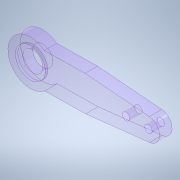
# Autodesk Inventor part: 後ろウィング中間ver2根元
Saved by Autodesk Inventor 2020.2 (Build 242310000, 310)
## iProperties
Created: 2020-05-07
Part Number: 後ろウィング中間ver2根元
Material: ポリカーボネート、クリア
Document SubType Name: Modeling
Designer: mozar
Density: 1.2 g/cm^3
Appearance: ポリカーボネート - クリア
Author: mozar
Autodesk Inventor part; units mm, degrees
ref_plane "YZ Plane" through (0, 0, 0) normal (1, 0, 0) x (0, 1, 0)
ref_plane "XZ Plane" through (0, 0, 0) normal (0, 1, 0) x (-1, 0, 0)
ref_plane "XY Plane" through (0, 0, 0) normal (0, 0, 1) x (1, 0, 0)
sketch "スケッチ1" plane through (0, 0, 0) normal (0, 0, 1) x (1, 0, 0)
  line L0 (-101.5, 47.999998) -> (108.5, 47.999998)
  circle A0 centre (111.885049, -39.000002) radius 4
  circle A1 centre (191.876682, -37.842982) radius 4
  circle A2 centre (111.885049, -39.000002) radius 7
  circle A3 centre (191.876682, -37.842982) radius 7
  line L1 (191.876682, -37.842982) -> (111.885049, -39.000002) construction
  line L2 (191.775442, -30.843714) -> (111.78381, -32.000734)
  line L3 (111.986288, -45.99927) -> (191.977921, -44.84225)
  arc A4 (191.977921, -44.84225) -> (191.775442, -30.843714) centre (191.876682, -37.842982) ccw
  arc A5 (111.78381, -32.000734) -> (111.986288, -45.99927) centre (111.885049, -39.000002) ccw
  line L4 (193.542302, -31.044032) -> (241.704818, -42.842982)
  circle A6 centre (234.566446, -71.981335) radius 30
  line L5 (262.587356, -82.697145) -> (213.725294, -50.402494)
  line L6 (213.725294, -50.402494) -> (190.211062, -44.641931)
  line L7 (264.566446, -121.542906) -> (264.566446, -63.2267)
  line L8 (111.885049, -39.000002) -> (111.885049, 40.999998) construction
  line L9 (118.885049, -39.000002) -> (118.885049, 40.999998)
  line L10 (104.885049, 40.999998) -> (104.885049, -39.000002)
  arc A7 (104.885049, -39.000002) -> (118.885049, -39.000002) centre (111.885049, -39.000002) ccw
  arc A8 (118.885049, 40.999998) -> (104.885049, 40.999998) centre (111.885049, 40.999998) ccw
  circle A9 centre (58.238326, 51.481995) radius 30
  line L11 (113.558078, 34.202868) -> (65.408448, 22.351438)
  line L12 (28.441083, 47.999998) -> (86.70408, 42.010942)
  line L13 (86.70408, 42.010942) -> (110.21202, 47.797128)
  circle A10 centre (113.5, -20.000002) radius 68
  line L14 (315.327237, -100.585467) -> (70.600424, 104.764712)
  line L15 (253.850074, -49.000002) -> (111.885049, -39.000002)
  arc A11 (93.592427, -27.104845) -> (135.370976, -5.924402) centre (95.060351, 21.794105) ccw
  arc A12 (135.370976, -5.924402) -> (135.847591, -3.671647) centre (132.898992, -4.224609) ccw
  arc A13 (135.847591, -3.671647) -> (83.183341, 18.55647) centre (102.157897, -9.989602) ccw
  line L16 (111.885049, -39.000002) -> (112.74718, 40.995353) construction
  line L17 (118.884642, -39.075438) -> (119.746773, 40.919916)
  line L18 (105.747586, 41.070789) -> (104.885455, -38.924565)
  arc A14 (104.885455, -38.924565) -> (118.884642, -39.075438) centre (111.885049, -39.000002) ccw
  arc A15 (119.746773, 40.919916) -> (105.747586, 41.070789) centre (112.74718, 40.995353) ccw
  line L19 (164.994898, 47.999998) -> (164.994898, 25.999998)
  line L20 (164.994898, 25.999998) -> (327.494898, -102.000002)
  circle A16 centre (116.292557, -40.000002) radius 68
  circle A17 centre (-98.885049, -0.000002) radius 67.5
  line L21 (321.363327, -8.500986) -> (-152.668056, 78.49822)
  line L22 (104.889695, -3) -> (104.889695, 0)
  line L23 (104.889695, -3) -> (64.444342, -3)
  line L24 (72.06562, 0) -> (104.889695, 0)
  circle A18 centre (83.376901, -17.5) radius 13.85
  line L25 (198.510163, -35.607603) -> (190.779084, -12.665641)
  line L26 (185.2432, -40.07836) -> (169.408184, 6.912016)
  circle A19 centre (197.837392, 16.492211) radius 30
  line L27 (190.779084, -12.665641) -> (191.876682, 45.89408)
  circle A20 centre (191.876682, -37.842982) radius 83.737062
  line L28 (191.876682, 45.89408) -> (191.876682, -37.842982)
  line L29 (96.889695, -3) -> (96.889695, -6)
  line L30 (96.889695, -6) -> (87.889695, -6)
  line L31 (87.889695, -6) -> (87.889695, -3)
  line L32 (76.444342, -3) -> (76.444342, -6)
  line L33 (76.444342, -6) -> (67.444342, -6)
  line L34 (67.444342, -6) -> (67.444342, -3)
  line L35 (99.889695, -3) -> (99.889695, 0)
  line L36 (99.889695, 0) -> (84.889695, 0)
  line L37 (84.889695, 0) -> (84.889695, -3)
  line L38 (79.444342, -3) -> (79.444342, 0)
  line L39 (79.444342, 0) -> (64.444342, 0)
  line L40 (64.444342, 0) -> (64.444342, -3)
  line L41 (64.444342, 0) -> (59.444342, 0)
  line L42 (59.444342, 0) -> (59.444342, -3)
  line L43 (59.444342, -3) -> (64.444342, -3)
  line L44 (59.444342, -3) -> (59.444342, -6)
  circle A21 centre (111.885049, -39.000002) radius 1.5
  circle A22 centre (111.885049, -39.000002) radius 9
  circle A23 centre (111.885049, -39.000002) radius 10
  circle A24 centre (111.885049, -39.000002) radius 15
  line L45 (121.057661, -50.868582) -> (142.927269, -50.552254)
  line L46 (121.057661, -50.868582) -> (127.651316, -45.772687)
  line L47 (127.651316, -45.772687) -> (126.808053, -37.482129)
  line L48 (124.15135, -30.366471) -> (104.889695, -3)
  line L49 (101.060181, -49.383751) -> (59.444342, -6)
  circle A25 centre (95.889695, -6) radius 1
  circle A26 centre (88.889695, -6) radius 1
  circle A27 centre (95.889695, -3) radius 1
  circle A28 centre (88.889695, -3) radius 1
  circle A29 centre (100.889695, -3) radius 1
  circle A30 centre (83.889695, -3) radius 1
  circle A31 centre (80.444342, -3) radius 1
  circle A32 centre (75.444342, -6) radius 1
  circle A33 centre (68.444342, -6) radius 1
  circle A34 centre (75.444342, -3) radius 1
  circle A35 centre (68.444342, -3) radius 1
  circle A36 centre (63.444342, -3) radius 1
  line L50 (189.021336, -49.498324) -> (211.692496, -55.05235)
  line L51 (211.692496, -55.05235) -> (259.830429, -86.868398)
  circle A37 centre (191.876682, -37.842982) radius 8
  circle A38 centre (191.876682, -37.842982) radius 13
  line L52 (198.876682, -21.280236) -> (198.876682, -52.125839)
  circle A39 centre (194.376682, -52.125839) radius 4.5
  circle A40 centre (194.376682, -52.125839) radius 1.5
  circle A41 centre (177.559161, -35.549813) radius 1.5
  circle A42 centre (194.376682, -52.125839) radius 4.5
  circle A43 centre (177.559161, -35.549813) radius 4.5
  circle A44 centre (191.876682, -37.842982) radius 1.5
  circle A45 centre (191.876682, -37.842982) radius 4.5
  line L53 (198.809292, -51.349976) -> (196.309292, -37.06712)
  line L54 (192.588353, -33.399614) -> (178.270831, -31.106451)
  circle A46 centre (181.698049, -48.169909) radius 1.5
  circle A47 centre (181.698049, -48.169909) radius 4.5
  line L55 (193.036341, -56.421591) -> (180.357708, -52.465661)
  line L56 (177.422132, -49.57224) -> (173.283242, -36.952144)
  point P0 (0, 0)
  point P1 (0, 0)
  point P2 (151.880865, -38.421492)
  point P3 (111.885049, 0.999998)
  point P4 (105.885049, -0.000002)
  point P5 (105.885049, -0.000002)
  point P6 (23.732778, -42.728965)
  point P7 (112.316114, 0.997675)
  point P8 (99.889695, -1.5)
  point P9 (76.444342, -4.5)
  point P10 (74.444342, -6)
  point P11 (69.444342, -6)
  point P12 (69.444342, -3)
  point P13 (74.444342, -3)
  point P14 (82.889695, -3)
  point P15 (81.444342, -3)
  point P16 (62.444342, -3)
  point P17 (101.889695, -3)
  point P18 (89.889695, -3)
  point P19 (94.889695, -3)
  point P20 (94.889695, -6)
  point P21 (89.889695, -6)
  point P22 (118.961603, -31.934425)
  point P23 (118.924491, -31.897449)
  point P24 (118.962007, -31.896907)
  point P25 (119.12697, -45.895985)
  point P26 (104.885049, -3)
  point P27 (104.885049, -31.858573)
  point P28 (117.642551, -45.917456)
  point P29 (175.94693, -45.074126)
  point P30 (198.871572, -51.911454)
  point P31 (198.876682, -51.912706)
  point P32 (198.876682, -46.764852)
  point P33 (193.972807, -45.563491)
  point P34 (184.006402, -36.408166)
  point P35 (182.178049, -30.982533)
  point P36 (117.440072, -31.91892)
  point P37 (180.360015, -43.873438)
  point P38 (180.33295, -43.821464)
  point P39 (180.497374, -43.833046)
  dimension "d27" = 167.47412
  dimension "d70" = 9
  dimension "d0" = 8
  dimension "d1" = 8
  dimension "d2" = 3
  dimension "d3" = 3
  dimension "d4" = 80
  dimension "d5" = 14
  dimension "d6" = 14
  dimension "d7" = 60
  dimension "d8" = 14
  dimension "d9" = 60
  dimension "d10" = 14
  dimension "d11" = 6
  dimension "d12" = 40
  dimension "d13" = 13.271
  dimension "d14" = 14
  dimension "d15" = 10
  dimension "d16" = 5
  dimension "d17" = 22
  dimension "d18" = 150
  dimension "d19" = 162.5
  dimension "d20" = 0
  dimension "d21" = 136
  dimension "d22" = 136
  dimension "d23" = 135
  dimension "d24" = 38.2272
  dimension "d25" = 25
  dimension "d26" = 60
  dimension "d28" = 5
  dimension "d29" = 3
  dimension "d30" = 5
  dimension "d31" = 3
  dimension "d32" = 3
  dimension "d33" = 5
  dimension "d34" = 1
  dimension "d35" = 5
  dimension "d36" = 5
  dimension "d37" = 2
  dimension "d38" = 2
  dimension "d39" = 2
  dimension "d40" = 2
  dimension "d41" = 2
  dimension "d42" = 2
  dimension "d43" = 2
  dimension "d44" = 2
  dimension "d45" = 2
  dimension "d46" = 2
  dimension "d47" = 2
  dimension "d48" = 2
  dimension "d49" = 5
  dimension "d50" = 1
  dimension "d51" = 6
  dimension "d57" = 3
  dimension "d58" = 3
  dimension "d59" = 3
  dimension "d60" = 3
  dimension "d61" = 3
  dimension "d62" = 3
  dimension "d65" = 109.028
  dimension "d67" = 3
  dimension "d68" = 9
  dimension "d69" = 72.2057
  dimension "d71" = 54.514
  constraints: 118 end point, 59 tangent, 46 centre point, 45 point on circle, 16 vertical, 8 coincident, 8 point on line, 7 equal length, 7 horizontal, 5 midpoint, 5 parallel, 1 concentric, 1 perpendicular, 1 vertical alignment, 29 other
  measures "d0" diameter of A0
  measures "d1" diameter of A1
  measures "d2" radial gap between concentric circles of A0 A2
  measures "d3" radial gap between concentric circles of A1 A3
  measures "d4" distance of L1.start L1.end
  measures "d5" diameter of A5
  measures "d6" distance from line of L4 L5.end
  measures "d7" diameter of A6
  measures "d8" diameter of A8
  measures "d9" diameter of A9
  measures "d10" distance from line of L11 L12.end
  measures "d11" horizontal distance of L1.end point (105.885, 0)
  measures "d12" angle of L14 L0
  measures "d14" diameter of A15
  measures "d15" vertical distance of L15.start L1.end
  measures "d16" vertical distance of L1.start L4.end
  measures "d17" distance of L19.start L19.end
  measures "d18" vertical distance of L19.start L20.end
  measures "d19" distance from line of L19 L20.end
  measures "d20" distance from line of L19.start L0
  measures "d21" diameter of A10
  measures "d22" diameter of A16
  measures "d23" diameter of A17
  measures "d24" angle of L0 L20
  measures "d25" distance from line of L5.start L20
  measures "d26" diameter of A19
  measures "d28" distance between parallel lines of L35 L22
  measures "d29" distance of L41.end L42.end
  measures "d30" distance of L42.end L40.end
  measures "d31" distance of L42.end L44.end
  measures "d32" diameter of A21
  measures "d33" radial gap between concentric circles of A0 A22
  measures "d34" radial gap between concentric circles of A22 A23
  measures "d35" radial gap between concentric circles of A23 A24
  measures "d36" distance between parallel lines of L3 L45
  measures "d37" diameter of A25
  measures "d38" diameter of A26
  measures "d39" diameter of A27
  measures "d40" diameter of A28
  measures "d41" diameter of A29
  measures "d42" diameter of A30
  measures "d43" diameter of A31
  measures "d44" diameter of A32
  measures "d45" diameter of A33
  measures "d46" diameter of A34
  measures "d47" diameter of A35
  measures "d48" diameter of A36
  measures "d49" distance between parallel lines of L6 L50
  measures "d50" radial gap between concentric circles of A3 A37
  measures "d51" radial gap between concentric circles of A3 A38
  measures "d57" diameter of A40
  measures "d58" diameter of A41
  measures "d59" radial gap between concentric circles of A40 A42
  measures "d60" radial gap between concentric circles of A41 A43
  measures "d61" diameter of A44
  measures "d62" radial gap between concentric circles of A44 A45
  measures "d67" diameter of A46
  measures "d68" diameter of A47
  measures "d69" angle of L26 L2
sketch "スケッチ1 outline for 押し出し1" plane through (0, 0, 0) normal (0, 0, 1) x (1, 0, 0)
  arc A0 (117.440072, -31.91892) -> (117.642551, -45.917456) centre (111.885049, -39.000002) ccw
  line L0 (182.178049, -30.982533) -> (117.440072, -31.91892)
  line L1 (117.642551, -45.917456) -> (175.94693, -45.074126)
  line L2 (184.006402, -36.408166) -> (182.178049, -30.982533)
  line L3 (175.94693, -45.074126) -> (177.422132, -49.57224)
  arc A1 (193.972807, -45.563491) -> (184.006402, -36.408166) centre (191.876682, -37.842982) cw
  arc A2 (177.422132, -49.57224) -> (180.357708, -52.465661) centre (181.698047, -48.169912) ccw
  line L4 (198.876682, -46.764852) -> (193.972807, -45.563491)
  line L5 (180.357708, -52.465661) -> (193.036341, -56.421591)
  line L6 (198.876682, -51.912706) -> (198.876682, -46.764852)
  arc A3 (193.036341, -56.421591) -> (198.871572, -51.911454) centre (194.376682, -52.125838) ccw
  line L7 (198.871572, -51.911454) -> (198.876682, -51.912706)
  arc A4 (180.360015, -43.873438) -> (180.33295, -43.821464) centre (191.876682, -37.842982) cw
  arc A5 (180.497374, -43.833046) -> (180.360015, -43.873438) centre (181.698049, -48.169909) ccw
  line L8 (180.33295, -43.821464) -> (180.497374, -43.833046)
  circle A6 centre (181.698049, -48.169909) radius 1.5
  circle A7 centre (194.376682, -52.125839) radius 1.5
  circle A8 centre (177.559161, -35.549813) radius 1.5
extrude "押し出し1" add sketch "スケッチ1 outline for 押し出し1" against normal blind 5
hole "穴1" at (105.885049, -0.000002, 0) at (113.5, -20.000002, 0) at (23.732778, -42.728965, 0) at (-98.885049, -0.000002, 0) at (111.885049, -39.000002, 0) direction (0, 0, -1) diameter 8.05 depth 12 tip angle 118
sketch "スケッチ2" plane through (0, 0, 0) normal (0, 0, 1) x (1, 0, 0)
  circle A0 centre (111.885049, -39.000002) radius 4.025
  line L0 (182.178049, -30.982533) -> (117.440072, -31.91892)
  arc A1 (117.440072, -31.91892) -> (117.642551, -45.917456) centre (111.885049, -39.000002) ccw
  line L1 (117.642551, -45.917456) -> (175.94693, -45.074126)
  line L2 (175.94693, -45.074126) -> (177.422132, -49.57224)
  arc A2 (177.422132, -49.57224) -> (180.357708, -52.465661) centre (181.698049, -48.169909) ccw
  line L3 (180.357708, -52.465661) -> (193.036341, -56.421591)
  arc A3 (193.036341, -56.421591) -> (198.871572, -51.911454) centre (194.376682, -52.125839) ccw
  line L4 (198.871572, -51.911454) -> (198.876682, -51.912706)
  line L5 (198.876682, -51.912706) -> (198.876682, -46.764852)
  line L6 (198.876682, -46.764852) -> (193.972807, -45.563491)
  arc A4 (184.006402, -36.408166) -> (193.972807, -45.563491) centre (191.876682, -37.842982) ccw
  line L7 (184.006402, -36.408166) -> (182.178049, -30.982533)
  circle A5 centre (194.376682, -52.125839) radius 1.5
  circle A6 centre (177.559161, -35.549813) radius 1.5
  circle A7 centre (181.698049, -48.169909) radius 1.5
  arc A8 (180.497374, -43.833046) -> (180.360015, -43.873438) centre (181.698049, -48.169909) ccw
  arc A9 (180.33295, -43.821464) -> (180.360015, -43.873438) centre (191.876682, -37.842982) ccw
  line L8 (180.33295, -43.821464) -> (180.497374, -43.833046)
  circle A10 centre (191.876682, -37.842982) radius 4.025
  arc A11 (193.542302, -31.044032) -> (185.672866, -34.600657) centre (191.876682, -37.842982) ccw
  line L9 (185.672866, -34.600657) -> (178.725027, -47.894548)
  line L10 (178.725027, -47.894548) -> (183.433896, -52.404723)
  line L11 (183.433896, -52.404723) -> (188.697561, -50.51843)
  line L12 (188.697561, -50.51843) -> (189.57433, -47.017413)
  line L13 (189.57433, -47.017413) -> (184.168816, -48.954539)
  line L14 (184.168816, -48.954539) -> (183.179583, -48.007047)
  line L15 (183.179583, -48.007047) -> (184.569151, -45.348268)
  line L16 (184.569151, -45.348268) -> (191.263493, -44.899758)
  line L17 (191.263493, -44.899758) -> (213.725294, -50.402494)
  line L18 (213.725294, -50.402494) -> (262.587356, -82.697145)
  arc A12 (262.587356, -82.697145) -> (241.704818, -42.842982) centre (234.566446, -71.981335) ccw
  line L19 (241.704818, -42.842982) -> (193.542302, -31.044032)
  circle A13 centre (191.876682, -37.842982) radius 16.83226
  circle A14 centre (177.559161, -35.549813) radius 1.5
  circle A15 centre (178.961677, -35.529526) radius 4.5
  line L20 (182.178049, -30.982533) -> (117.440072, -31.91892)
  circle A16 centre (178.961677, -35.529526) radius 1.5
  circle A17 centre (166.904743, -40.704444) radius 4.5
  circle A18 centre (166.904743, -40.704444) radius 1.5
  line L21 (191.876682, -37.842982) -> (178.961677, -35.529526)
  line L22 (178.961677, -35.529526) -> (166.904743, -40.704444)
  point P0 (0, 0)
  point P1 (0, 0)
  dimension "d82" = 9
  dimension "d83" = 3
  dimension "d84" = 9
  dimension "d85" = 3
  constraints: 26 end point, 7 centre point, 4 point on circle, 3 coincident, 3 tangent, 1 equal length, 1 vertical, 70 other
  measures "d82" diameter of A15
  measures "d83" diameter of A16
  measures "d84" diameter of A17
  measures "d85" diameter of A18
sketch "スケッチ3" plane through (0, 0, 0) normal (0, 0, 1) x (1, 0, 0)
  circle A0 centre (191.876682, -37.842982) radius 4.025
  line L0 (185.418769, -40.543975) -> (191.206612, -54.382359)
  line L1 (191.206612, -54.382359) -> (196.207213, -53.344445)
  line L2 (196.207213, -53.344445) -> (200.870857, -49.312531)
  line L3 (200.870857, -49.312531) -> (194.016935, -50.735116)
  line L4 (194.016935, -50.735116) -> (192.175534, -46.332438)
  line L5 (192.175534, -46.332438) -> (193.402436, -45.42376)
  line L6 (193.402436, -45.42376) -> (213.725294, -50.402494)
  line L7 (213.725294, -50.402494) -> (262.587356, -82.697145)
  arc A1 (262.587356, -82.697145) -> (241.704818, -42.842982) centre (234.566446, -71.981335) ccw
  line L8 (241.704818, -42.842982) -> (193.542302, -31.044032)
  arc A2 (193.542302, -31.044032) -> (185.418769, -40.543975) centre (191.876682, -37.842982) ccw
  point P0 (0, 0)
  point P1 (0, 0)
  constraints: 18 end point, 4 point on circle, 3 centre point
sketch "スケッチ4" plane through (0, 0, 0) normal (0, 0, 1) x (1, 0, 0)
  line L0 (194.745121, -45.752694) -> (213.725294, -50.402494)
  line L1 (213.725294, -50.402494) -> (262.587356, -82.697145)
  arc A0 (262.587356, -82.697145) -> (241.704818, -42.842982) centre (234.566446, -71.981335) ccw
  line L2 (241.704818, -42.842982) -> (193.542302, -31.044032)
  arc A1 (193.542302, -31.044032) -> (185.418769, -40.543975) centre (191.876682, -37.842982) ccw
  line L3 (185.418769, -40.543975) -> (191.206612, -54.382359)
  line L4 (191.206612, -54.382359) -> (195.655899, -53.216469)
  line L5 (195.655899, -53.216469) -> (195.656069, -53.216296)
  arc A2 (195.656069, -53.216296) -> (195.656308, -53.216236) centre (194.922022, -50.307486) ccw
  line L6 (195.656308, -53.216236) -> (198.568436, -51.556289)
  line L7 (198.568436, -51.556289) -> (199.758723, -49.040078)
  line L8 (199.758723, -49.040078) -> (195.762722, -50.087189)
  arc A3 (194.586681, -49.505705) -> (195.762722, -50.087189) centre (195.50924, -49.119849) ccw
  line L9 (194.586681, -49.505705) -> (193.584616, -47.109828)
  arc A4 (194.745121, -45.752694) -> (193.584616, -47.109828) centre (194.507175, -46.723972) ccw
  circle A5 centre (191.876682, -37.842982) radius 4.025
  circle A6 centre (111.885049, -39.000002) radius 4.025
  line L10 (182.178049, -30.982533) -> (117.440072, -31.91892)
  arc A7 (117.440072, -31.91892) -> (117.642551, -45.917456) centre (111.885049, -39.000002) ccw
  line L11 (117.642551, -45.917456) -> (175.94693, -45.074126)
  line L12 (175.94693, -45.074126) -> (177.422132, -49.57224)
  arc A8 (177.422132, -49.57224) -> (180.357708, -52.465661) centre (181.698049, -48.169909) ccw
  line L13 (180.357708, -52.465661) -> (193.036341, -56.421591)
  arc A9 (193.036341, -56.421591) -> (198.871572, -51.911454) centre (194.376682, -52.125839) ccw
  line L14 (198.871572, -51.911454) -> (198.876682, -51.912706)
  line L15 (198.876682, -51.912706) -> (198.876682, -46.764852)
  line L16 (198.876682, -46.764852) -> (193.972807, -45.563491)
  arc A10 (184.006402, -36.408166) -> (193.972807, -45.563491) centre (191.876682, -37.842982) ccw
  line L17 (184.006402, -36.408166) -> (182.178049, -30.982533)
  circle A11 centre (194.376682, -52.125839) radius 1.5
  circle A12 centre (177.559161, -35.549813) radius 1.5
  circle A13 centre (181.698049, -48.169909) radius 1.5
  arc A14 (180.497374, -43.833046) -> (180.360015, -43.873438) centre (181.698049, -48.169909) ccw
  arc A15 (180.33295, -43.821464) -> (180.360015, -43.873438) centre (191.876682, -37.842982) ccw
  line L18 (180.33295, -43.821464) -> (180.497374, -43.833046)
  line L19 (191.876682, -37.842982) -> (111.885049, -39.000002) construction
  line L20 (191.775442, -30.843714) -> (111.78381, -32.000734)
  line L21 (111.986288, -45.99927) -> (191.977921, -44.84225)
  arc A16 (191.977921, -44.84225) -> (191.775442, -30.843714) centre (191.876682, -37.842982) ccw
  arc A17 (111.78381, -32.000734) -> (111.986288, -45.99927) centre (111.885049, -39.000002) ccw
  circle A18 centre (178.961677, -35.529526) radius 4.5
  circle A19 centre (178.961677, -35.529526) radius 1.5
  circle A20 centre (183.157555, -46.799925) radius 1.5
  circle A21 centre (183.157555, -46.799925) radius 4.5
  line L22 (182.178049, -30.982533) -> (117.440072, -31.91892)
  line L23 (197.834841, -41.517261) -> (208.997311, -23.41636)
  line L24 (197.834841, -41.517261) -> (181.973255, -67.238185)
  circle A22 centre (170.35293, -38.154307) radius 4.5
  circle A23 centre (170.35293, -38.154307) radius 1.5
  line L25 (188.270523, -60.320544) -> (180.805974, -42.473256)
  arc A24 (194.73203, -26.18764) -> (180.805974, -42.473256) centre (191.876682, -37.842982) ccw
  line L26 (194.73203, -26.18764) -> (242.894547, -37.986589)
  arc A25 (264.570959, -90.00158) -> (242.894547, -37.986589) centre (234.566446, -71.981335) ccw
  line L27 (264.570959, -90.00158) -> (211.692496, -55.05235)
  line L28 (208.863654, -41.485411) -> (202.414104, -55.119458)
  line L29 (202.414104, -55.119458) -> (198.735697, -57.216192)
  line L30 (198.735697, -57.216192) -> (198.256714, -57.703764)
  line L31 (198.256714, -57.703764) -> (188.270523, -60.320544)
  line L32 (189.614177, -50.574943) -> (183.680676, -51.269416)
  arc A26 (184.006402, -36.408166) -> (193.972807, -45.563491) centre (191.876682, -37.842982) ccw
  point P0 (0, 0)
  point P1 (0, 0)
  point P2 (151.880865, -38.421492)
  point P3 (186.913184, -44.11703)
  point P4 (186.913184, -44.11703)
  point P5 (179.020383, -45.029671)
  dimension "d90" = 9
  dimension "d86" = 14
  dimension "d87" = 9
  dimension "d88" = 3
  dimension "d89" = 3
  dimension "d91" = 122.49
  dimension "d92" = 9
  dimension "d93" = 3
  dimension "d94" = 5
  dimension "d95" = 7
  constraints: 48 end point, 20 point on circle, 15 centre point, 7 tangent, 3 coincident, 3 point on line, 1 collinear, 1 equal radius, 1 midpoint, 1 parallel, 50 other
  measures "d86" diameter of A17
  measures "d87" diameter of A18
  measures "d88" diameter of A19
  measures "d89" diameter of A20
  measures "d91" angle of L23 L11
  measures "d92" diameter of A22
  measures "d93" diameter of A23
  measures "d94" distance between parallel lines of L3 L25
  measures "d95" distance of L32.start point (186.913, -44.117)
extrude "押し出し2" cut sketch "スケッチ4" against normal blind 10 contours L0 L24 A2 L9 A4 | A4 L9 A2 L24 L3 L21 A10 L16 | L0 L15 L8 A2 L24 | L24 L9 A2 | A2 L8 A3 L9 L24 | L9 L24 A2 | L21 L3 A10 | L15 L7 L6 A2 L8 | A2 L6 A11 L24 L9 A3 L8 | A2 A11 L4 L3 L24 | L15 L14 A9 L13 L24 L3 L4 A11 A2 L6 L7 | L24 L13 L25 L32 L3 | A2 L6 | A2 L4 A11 | L25 L13 A8 L12 L21 A21 L32 picked at (195.430042, -53.271235)
extrude "押し出し3" add sketch "スケッチ4" against normal blind 5 contours A20 A13 | A13 L25 A20 | A13 L25 | A19 A12 | A12 A19 picked at (182.922726, -47.847814)
hole "穴2" at (183.157555, -46.799925, 0) at (178.961677, -35.529526, 0) at (170.35293, -38.154307, 0) direction (0, 0, -1) diameter 3 depth 12 tip angle 118
sketch "スケッチ5" plane through (0, 0, 0) normal (0, 0, 1) x (1, 0, 0)
  circle A0 centre (178.961677, -35.529526) radius 1.5
  circle A1 centre (183.157555, -46.799925) radius 1.5
  circle A2 centre (170.35293, -38.154307) radius 1.5
  line L0 (189.614177, -50.574943) -> (186.913184, -44.11703)
  arc A3 (184.006402, -36.408166) -> (186.913184, -44.11703) centre (191.876682, -37.842982) ccw
  line L1 (184.006402, -36.408166) -> (182.178049, -30.982533)
  line L2 (182.178049, -30.982533) -> (117.440072, -31.91892)
  arc A4 (117.440072, -31.91892) -> (117.642551, -45.917456) centre (111.885049, -39.000002) ccw
  line L3 (117.642551, -45.917456) -> (179.020383, -45.029671)
  arc A5 (179.020383, -45.029671) -> (183.680676, -51.269416) centre (183.157555, -46.799925) ccw
  line L4 (183.680676, -51.269416) -> (189.614177, -50.574943)
  circle A6 centre (111.885049, -39.000002) radius 4.025
  arc A7 (180.497374, -43.833046) -> (180.360015, -43.873438) centre (181.698049, -48.169909) ccw
  arc A8 (180.33295, -43.821464) -> (180.360015, -43.873438) centre (191.876682, -37.842982) ccw
  line L5 (180.33295, -43.821464) -> (180.497374, -43.833046)
  circle A9 centre (111.885049, -39.000002) radius 4.025
  circle A10 centre (111.885049, -39.000002) radius 6
  point P0 (0, 0)
  dimension "d107" = 12
  constraints: 1 centre point, 1 coincident
  measures "d107" diameter of A10
extrude "押し出し4" cut sketch "スケッチ5" against normal blind 1 contours A10
sketch "スケッチ6" plane through (0, 0, 0) normal (0, 0, 1) x (1, 0, 0)
  circle A0 centre (111.885049, -39.000002) radius 6
  circle A1 centre (178.961677, -35.529526) radius 1.5
  circle A2 centre (183.157555, -46.799925) radius 1.5
  circle A3 centre (170.35293, -38.154307) radius 1.5
  line L0 (189.614177, -50.574943) -> (186.913184, -44.11703)
  arc A4 (184.006402, -36.408166) -> (186.913184, -44.11703) centre (191.876682, -37.842982) ccw
  line L1 (184.006402, -36.408166) -> (182.178049, -30.982533)
  line L2 (182.178049, -30.982533) -> (117.440072, -31.91892)
  arc A5 (117.440072, -31.91892) -> (117.642551, -45.917456) centre (111.885049, -39.000002) ccw
  line L3 (117.642551, -45.917456) -> (179.020383, -45.029671)
  arc A6 (179.020383, -45.029671) -> (183.680676, -51.269416) centre (183.157555, -46.799925) ccw
  line L4 (183.680676, -51.269416) -> (189.614177, -50.574943)
  arc A7 (180.497374, -43.833046) -> (180.360015, -43.873438) centre (181.698049, -48.169909) ccw
  arc A8 (180.33295, -43.821464) -> (180.360015, -43.873438) centre (191.876682, -37.842982) ccw
  line L5 (180.33295, -43.821464) -> (180.497374, -43.833046)
  circle A9 centre (170.35293, -38.154307) radius 1.5
  circle A10 centre (170.35293, -38.154307) radius 4.5
  circle A11 centre (191.876682, -37.842982) radius 7
  line L6 (184.006402, -36.408166) -> (185.2432, -40.07836)
  line L7 (188.222991, -43.813789) -> (160.136439, -26.626904)
  line L8 (160.136439, -26.626904) -> (159.163513, -26.031546)
  circle A12 centre (166.361389, -35.71178) radius 4.5
  circle A13 centre (166.361389, -35.71178) radius 1.5
  line L9 (182.178049, -30.982533) -> (117.440072, -31.91892)
  circle A14 centre (175.744086, -41.453294) radius 4.5
  point P0 (0, 0)
  point P1 (178.464745, -45.037708)
  point P2 (173.128236, -45.114896)
  point P3 (167.598953, -31.193409)
  point P4 (184.919442, -41.792263)
  dimension "d110" = 9
  dimension "d111" = 14
  dimension "d112" = 9
  dimension "d113" = 3
  dimension "d114" = 9
  dimension "d115" = 11
  constraints: 6 end point, 6 tangent, 5 centre point, 3 coincident, 2 point on circle, 1 point on line
  measures "d110" diameter of A10
  measures "d111" diameter of A11
  measures "d112" diameter of A12
  measures "d113" diameter of A13
  measures "d114" diameter of A14
  measures "d115" distance of A12.centre A14.centre
extrude "押し出し5" add sketch "スケッチ6" against normal blind 5 contours A3 A12 | A12 A3 | L3 A14 | A7 A8 L5
hole "穴3" at (175.744086, -41.453294, 0) at (166.361389, -35.71178, 0) direction (0, 0, -1) diameter 3 depth 12 tip angle 118
extrude "押し出し6" cut sketch "スケッチ6" against normal blind 10 contours L7 L2 L1 A4
sketch "スケッチ7" plane through (0, 0, 0) normal (0, 0, 1) x (1, 0, 0)
  circle A0 centre (175.744086, -41.453294) radius 1.5
  circle A1 centre (166.361389, -35.71178) radius 1.5
  circle A2 centre (111.885049, -39.000002) radius 6
  circle A3 centre (183.157555, -46.799925) radius 1.5
  line L0 (186.913184, -44.11703) -> (189.614177, -50.574943)
  line L1 (189.614177, -50.574943) -> (183.680676, -51.269416)
  arc A4 (179.020383, -45.029671) -> (183.680676, -51.269416) centre (183.157555, -46.799925) ccw
  line L2 (179.020383, -45.029671) -> (178.464745, -45.037708)
  arc A5 (173.128236, -45.114896) -> (178.464745, -45.037708) centre (175.744086, -41.453294) ccw
  line L3 (173.128236, -45.114896) -> (117.642551, -45.917456)
  arc A6 (117.440072, -31.91892) -> (117.642551, -45.917456) centre (111.885049, -39.000002) ccw
  line L4 (117.440072, -31.91892) -> (167.598953, -31.193409)
  line L5 (167.598953, -31.193409) -> (184.919442, -41.792263)
  arc A7 (184.919442, -41.792263) -> (186.913184, -44.11703) centre (191.876682, -37.842982) ccw
  point P0 (0, 0)
sketch "スケッチ8" plane through (0, 0, 0) normal (0, 0, 1) x (1, 0, 0)
  line L0 (184.919442, -41.792263) -> (167.598953, -31.193409)
  line L1 (167.598953, -31.193409) -> (117.440072, -31.91892)
  arc A0 (117.440072, -31.91892) -> (117.642551, -45.917456) centre (111.885049, -39.000002) ccw
  line L2 (117.642551, -45.917456) -> (173.128236, -45.114896)
  arc A1 (173.128236, -45.114896) -> (178.464745, -45.037708) centre (175.744086, -41.453294) ccw
  line L3 (178.464745, -45.037708) -> (179.020383, -45.029671)
  arc A2 (179.020383, -45.029671) -> (183.680676, -51.269416) centre (183.157555, -46.799925) ccw
  line L4 (183.680676, -51.269416) -> (189.614177, -50.574943)
  line L5 (189.614177, -50.574943) -> (186.913184, -44.11703)
  arc A3 (184.919442, -41.792263) -> (186.913184, -44.11703) centre (191.876682, -37.842982) ccw
  circle A4 centre (183.157555, -46.799925) radius 1.5
  circle A5 centre (111.885049, -39.000002) radius 6
  circle A6 centre (166.361389, -35.71178) radius 1.5
  circle A7 centre (175.744086, -41.453294) radius 1.5
  circle A8 centre (111.885049, -39.000002) radius 4.025
  line L6 (191.876682, -37.842982) -> (111.885049, -39.000002)
  circle A9 centre (166.361389, -35.71178) radius 1.5
  circle A10 centre (166.361389, -35.71178) radius 4.5
  circle A11 centre (160.94376, -38.290404) radius 4.5
  circle A12 centre (160.94376, -38.290404) radius 1.5
  circle A13 centre (151.944701, -38.420568) radius 4.5
  circle A14 centre (151.944701, -38.420568) radius 1.5
  circle A15 centre (160.94376, -38.290404) radius 3
  circle A16 centre (151.944701, -38.420568) radius 3
  line L7 (165.530413, -31.28917) -> (151.113726, -33.997958)
  circle A17 centre (175.744086, -41.453294) radius 4.5
  line L8 (151.375872, -42.884472) -> (175.175257, -45.917198)
  arc A18 (117.440072, -31.91892) -> (117.642551, -45.917456) centre (111.885049, -39.000002) ccw
  circle A19 centre (111.885049, -39.000002) radius 9
  line L9 (161.421253, -42.764999) -> (112.840034, -47.949192)
  line L10 (161.291636, -33.80387) -> (112.580802, -30.026935)
  point P0 (0, 0)
  point P1 (0, 0)
  point P2 (169.312318, -45.170091)
  point P3 (166.296306, -31.212251)
  point P4 (134.111814, -45.67924)
  point P5 (168.71019, -31.873404)
  point P6 (166.296306, -31.212251)
  point P7 (133.909336, -31.680705)
  dimension "d128" = 9
  dimension "d129" = 3
  dimension "d130" = 9
  dimension "d131" = 3
  dimension "d132" = 6
  dimension "d133" = 6
  dimension "d134" = 9
  constraints: 22 end point, 19 centre point, 19 point on circle, 8 coincident, 7 tangent, 2 point on line, 24 other
  measures "d128" diameter of A11
  measures "d129" diameter of A12
  measures "d130" diameter of A13
  measures "d131" diameter of A14
  measures "d132" diameter of A15
  measures "d133" diameter of A16
  measures "d134" distance of A13.centre A11.centre
extrude "押し出し7" cut sketch "スケッチ8" against normal blind 10 contours A3 L5 L4 A2 L3 A17 L6 L0 | L6 A17 L0 | A17 L6 A10 L0 | A17 L6 | A17 A1 L6 | A10 L1 L0 | A6 | A10 L6 A11 | A17 L2 L8 L9 A11 A10 L6 | A10 L7 L10 L1 | A10 A11 L6 | A10 A11 L10 L7 | L2 L9 L8 | A7
sketch "スケッチ9" plane through (0, 0, 0) normal (0, 0, 1) x (1, 0, 0)
  line L0 (161.291636, -33.80387) -> (133.909336, -31.680705)
  line L1 (133.909336, -31.680705) -> (117.440072, -31.91892)
  arc A0 (117.440072, -31.91892) -> (117.642551, -45.917456) centre (111.885049, -39.000002) ccw
  line L2 (117.642551, -45.917456) -> (134.111814, -45.67924)
  line L3 (134.111814, -45.67924) -> (161.421253, -42.764999)
  arc A1 (161.421253, -42.764999) -> (161.291636, -33.80387) centre (160.94376, -38.290404) ccw
  circle A2 centre (111.885049, -39.000002) radius 6
  circle A3 centre (166.361389, -35.71178) radius 1.5
  circle A4 centre (166.361389, -35.71178) radius 3
  line L4 (160.94376, -38.290404) -> (151.944701, -38.420568)
  circle A5 centre (159.327217, -38.313786) radius 4.5
  line L5 (117.642551, -45.917456) -> (134.111814, -45.67924)
  line L6 (159.830351, -42.78557) -> (134.111814, -45.67924)
  line L7 (161.291636, -33.80387) -> (133.909336, -31.680705)
  line L8 (159.700806, -33.82932) -> (133.909336, -31.680705)
  circle A6 centre (150.328159, -38.443951) radius 4.5
  point P0 (0, 0)
  dimension "d146" = 6
  dimension "d147" = 9
  dimension "d148" = 9
  dimension "d149" = 9
  constraints: 6 end point, 3 centre point, 3 tangent, 2 point on circle, 2 point on line, 1 coincident, 1 other
  measures "d146" diameter of A4
  measures "d147" diameter of A5
  measures "d148" diameter of A6
  measures "d149" distance of A5.centre A6.centre
hole "穴5" at (159.327217, -38.313786, 0) at (150.328159, -38.443951, 0) direction (0, 0, -1) diameter 3 depth 12 tip angle 118
extrude "押し出し9" cut sketch "スケッチ9" against normal blind 10 contours A1 A4 A5 L8 L0 | A1 A4 | A4 A1 L3 L6 A5 picked at (164.393308, -36.270533)
equation "\"d9\" = d7"
equation "\"d26\" = d7"
equation "\"d71\" = 0.5 * d65"
